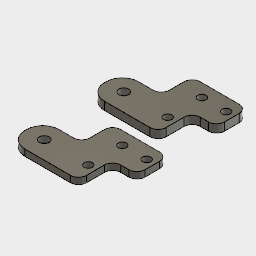
Y_Idler_Bracket_v2 (Autodesk Fusion 360 design; units mm, degrees)
Autodesk Fusion 360 part; units mm, degrees
sketch "Sketch1" plane through (0, 0, 0) normal (0, 1, 0) x (1, 0, 0)
  line L0 (-4, 15) -> (20, 15)
  line L1 (25, 10) -> (25, 1)
  line L2 (20, -4) -> (15, -4)
  line L3 (10, -9) -> (10, -20)
  line L4 (5, -25) -> (-23, -25)
  line L5 (-33, -15) -> (-33, -14)
  line L6 (-23, -4) -> (-14, -4)
  line L7 (-9, 1) -> (-9, 10)
  arc A0 (-4, 15) -> (-9, 10) centre (-4, 10) ccw
  arc A1 (-14, -4) -> (-9, 1) centre (-14, 1) ccw
  arc A2 (25, 10) -> (20, 15) centre (20, 10) ccw
  arc A3 (20, -4) -> (25, 1) centre (20, 1) ccw
  arc A4 (15, -4) -> (10, -9) centre (15, -9) ccw
  arc A5 (5, -25) -> (10, -20) centre (5, -20) ccw
  arc A6 (-23, -4) -> (-33, -14) centre (-23, -14) ccw
  arc A7 (-33, -15) -> (-23, -25) centre (-23, -15) ccw
  circle A8 centre (5, 7) radius 2.5
  circle A9 centre (20, 7) radius 2.5
  circle A10 centre (5, -14) radius 2.5
  circle A11 centre (-22.0816, -14) radius 3
  dimension "d1" = 5
  dimension "d2" = 10
  dimension "d3" = 5
  dimension "d4" = 5
  dimension "d5" = 5
  dimension "d6" = 6
  measures "d1" radius of A0
  measures "d2" radius of A6
  measures "d3" diameter of A8
  measures "d4" diameter of A9
  measures "d5" diameter of A10
  measures "d6" diameter of A11
extrude "Extrude1" add sketch "Sketch1" along normal blind 5 makes body 1
copy_body "CopyPasteBodies1" bodies 1 makes body 2
move_body "Move1" bodies 2 to x (1, 0, 0) y (0, 1, 0) z (0, 0, 1) at (0, 0, 49)
move_face "OffsetFaces1" offset -1 1 faces at (-0.5675, 5, 51.4696) on bodies 2
named bodies: "5mm", "4mm"
